Autodesk Fusion 360 part; units mm, degrees
(part 3 of 4)
  line L1272 (186.7093, 343.9871) -> (186.7093, 321.9621)
  line L1273 (186.7093, 321.9621) -> (208.7343, 321.9621)
  line L1274 (210.2343, 323.4621) -> (210.2343, 332.1121)
  line L1275 (210.2343, 332.1121) -> (213.3343, 332.1121)
  line L1276 (213.3343, 332.1121) -> (213.3343, 323.4621)
  line L1277 (214.8343, 321.9621) -> (236.8593, 321.9621)
  line L1278 (236.8593, 321.9621) -> (236.8593, 343.9871)
  line L1279 (235.3593, 345.4871) -> (226.7093, 345.4871)
  line L1280 (226.7093, 345.4871) -> (226.7093, 348.5871)
  line L1281 (226.7093, 348.5871) -> (235.3593, 348.5871)
  line L1282 (236.8593, 350.0871) -> (236.8593, 372.1121)
  line L1283 (236.8593, 372.1121) -> (214.8343, 372.1121)
  line L1284 (213.3343, 370.6121) -> (213.3343, 361.9621)
  line L1285 (213.3343, 361.9621) -> (210.2343, 361.9621)
  line L1286 (210.2343, 361.9621) -> (210.2343, 370.6121)
  line L1287 (208.7343, 372.1121) -> (186.7093, 372.1121)
  line L1288 (92.7953, 75.9662) -> (92.7953, 53.9412)
  line L1289 (94.2953, 52.4412) -> (102.9453, 52.4412)
  line L1290 (102.9453, 52.4412) -> (102.9453, 49.3412)
  line L1291 (102.9453, 49.3412) -> (94.2953, 49.3412)
  line L1292 (92.7953, 47.8412) -> (92.7953, 25.8162)
  line L1293 (92.7953, 25.8162) -> (114.8203, 25.8162)
  line L1294 (116.3203, 27.3162) -> (116.3203, 35.9662)
  line L1295 (116.3203, 35.9662) -> (119.4203, 35.9662)
  line L1296 (119.4203, 35.9662) -> (119.4203, 27.3162)
  line L1297 (120.9203, 25.8162) -> (142.9453, 25.8162)
  line L1298 (142.9453, 25.8162) -> (142.9453, 47.8412)
  line L1299 (141.4453, 49.3412) -> (132.7953, 49.3412)
  line L1300 (132.7953, 49.3412) -> (132.7953, 52.4412)
  line L1301 (132.7953, 52.4412) -> (141.4453, 52.4412)
  line L1302 (142.9453, 53.9412) -> (142.9453, 75.9662)
  line L1303 (142.9453, 75.9662) -> (120.9203, 75.9662)
  line L1304 (119.4203, 74.4662) -> (119.4203, 65.8162)
  line L1305 (119.4203, 65.8162) -> (116.3203, 65.8162)
  line L1306 (116.3203, 65.8162) -> (116.3203, 74.4662)
  line L1307 (114.8203, 75.9662) -> (92.7953, 75.9662)
  line L1308 (90.7952, 128.1162) -> (68.7702, 128.1162)
  line L1309 (67.2702, 126.6162) -> (67.2702, 117.9662)
  line L1310 (67.2702, 117.9662) -> (64.1702, 117.9662)
  line L1311 (64.1702, 117.9662) -> (64.1702, 126.6162)
  line L1312 (62.6702, 128.1162) -> (40.6452, 128.1162)
  line L1313 (40.6452, 128.1162) -> (40.6452, 106.0912)
  line L1314 (42.1452, 104.5912) -> (50.7952, 104.5912)
  line L1315 (50.7952, 104.5912) -> (50.7952, 101.4912)
  line L1316 (50.7952, 101.4912) -> (42.1452, 101.4912)
  line L1317 (40.6452, 99.9912) -> (40.6452, 77.9662)
  line L1318 (40.6452, 77.9662) -> (62.6702, 77.9662)
  line L1319 (64.1702, 79.4662) -> (64.1702, 88.1162)
  line L1320 (64.1702, 88.1162) -> (67.2702, 88.1162)
  line L1321 (67.2702, 88.1162) -> (67.2702, 79.4662)
  line L1322 (68.7702, 77.9662) -> (90.7952, 77.9662)
  line L1323 (90.7952, 77.9662) -> (90.7952, 99.9912)
  line L1324 (89.2952, 101.4912) -> (80.6452, 101.4912)
  line L1325 (80.6452, 101.4912) -> (80.6452, 104.5912)
  line L1326 (80.6452, 104.5912) -> (89.2952, 104.5912)
  line L1327 (90.7952, 106.0912) -> (90.7952, 128.1162)
  line L1328 (144.9453, 75.9662) -> (144.9453, 53.9412)
  line L1329 (146.4453, 52.4412) -> (155.0953, 52.4412)
  line L1330 (155.0953, 52.4412) -> (155.0953, 49.3412)
  line L1331 (155.0953, 49.3412) -> (146.4453, 49.3412)
  line L1332 (144.9453, 47.8412) -> (144.9453, 25.8162)
  line L1333 (144.9453, 25.8162) -> (166.9703, 25.8162)
  line L1334 (168.4703, 27.3162) -> (168.4703, 35.9662)
  line L1335 (168.4703, 35.9662) -> (171.5703, 35.9662)
  line L1336 (171.5703, 35.9662) -> (171.5703, 27.3162)
  line L1337 (173.0703, 25.8162) -> (195.0953, 25.8162)
  line L1338 (195.0953, 25.8162) -> (195.0953, 47.8412)
  line L1339 (193.5953, 49.3412) -> (184.9453, 49.3412)
  line L1340 (184.9453, 49.3412) -> (184.9453, 52.4412)
  line L1341 (184.9453, 52.4412) -> (193.5953, 52.4412)
  line L1342 (195.0953, 53.9412) -> (195.0953, 75.9662)
  line L1343 (195.0953, 75.9662) -> (173.0703, 75.9662)
  line L1344 (171.5703, 74.4662) -> (171.5703, 65.8162)
  line L1345 (171.5703, 65.8162) -> (168.4703, 65.8162)
  line L1346 (168.4703, 65.8162) -> (168.4703, 74.4662)
  line L1347 (166.9703, 75.9662) -> (144.9453, 75.9662)
  line L1348 (92.7953, 128.1162) -> (92.7953, 106.0912)
  line L1349 (94.2953, 104.5912) -> (102.9453, 104.5912)
  line L1350 (102.9453, 104.5912) -> (102.9453, 101.4912)
  line L1351 (102.9453, 101.4912) -> (94.2953, 101.4912)
  line L1352 (92.7953, 99.9912) -> (92.7953, 77.9662)
  line L1353 (92.7953, 77.9662) -> (114.8203, 77.9662)
  line L1354 (116.3203, 79.4662) -> (116.3203, 88.1162)
  line L1355 (116.3203, 88.1162) -> (119.4203, 88.1162)
  line L1356 (119.4203, 88.1162) -> (119.4203, 79.4662)
  line L1357 (120.9203, 77.9662) -> (142.9453, 77.9662)
  line L1358 (142.9453, 77.9662) -> (142.9453, 99.9912)
  line L1359 (141.4453, 101.4912) -> (132.7953, 101.4912)
  line L1360 (132.7953, 101.4912) -> (132.7953, 104.5912)
  line L1361 (132.7953, 104.5912) -> (141.4453, 104.5912)
  line L1362 (142.9453, 106.0912) -> (142.9453, 128.1162)
  line L1363 (142.9453, 128.1162) -> (120.9203, 128.1162)
  line L1364 (119.4203, 126.6162) -> (119.4203, 117.9662)
  line L1365 (119.4203, 117.9662) -> (116.3203, 117.9662)
  line L1366 (116.3203, 117.9662) -> (116.3203, 126.6162)
  line L1367 (114.8203, 128.1162) -> (92.7953, 128.1162)
  line L1368 (134.5593, 372.1123) -> (134.5593, 350.0873)
  line L1369 (136.0593, 348.5873) -> (144.7093, 348.5873)
  line L1370 (144.7093, 348.5873) -> (144.7093, 345.4873)
  line L1371 (144.7093, 345.4873) -> (136.0593, 345.4873)
  line L1372 (134.5593, 343.9873) -> (134.5593, 321.9623)
  line L1373 (134.5593, 321.9623) -> (156.5843, 321.9623)
  line L1374 (158.0843, 323.4623) -> (158.0843, 332.1123)
  line L1375 (158.0843, 332.1123) -> (161.1843, 332.1123)
  line L1376 (161.1843, 332.1123) -> (161.1843, 323.4623)
  line L1377 (162.6843, 321.9623) -> (184.7093, 321.9623)
  line L1378 (184.7093, 321.9623) -> (184.7093, 343.9873)
  line L1379 (183.2093, 345.4873) -> (174.5593, 345.4873)
  line L1380 (174.5593, 345.4873) -> (174.5593, 348.5873)
  line L1381 (174.5593, 348.5873) -> (183.2093, 348.5873)
  line L1382 (184.7093, 350.0873) -> (184.7093, 372.1123)
  line L1383 (184.7093, 372.1123) -> (162.6843, 372.1123)
  line L1384 (161.1843, 370.6123) -> (161.1843, 361.9623)
  line L1385 (161.1843, 361.9623) -> (158.0843, 361.9623)
  line L1386 (158.0843, 361.9623) -> (158.0843, 370.6123)
  line L1387 (156.5843, 372.1123) -> (134.5593, 372.1123)
  line L1388 (70.2592, 363.2374) -> (78.9092, 363.2374)
  line L1389 (80.4092, 364.7374) -> (80.4092, 374.2624)
  line L1390 (80.4092, 374.2624) -> (30.2592, 374.2624)
  line L1391 (30.2592, 374.2624) -> (30.2592, 364.7374)
  line L1392 (31.7592, 363.2374) -> (40.4092, 363.2374)
  line L1393 (40.4092, 363.2374) -> (40.4092, 360.1374)
  line L1394 (40.4092, 360.1374) -> (31.7592, 360.1374)
  line L1395 (30.2592, 358.6374) -> (30.2592, 349.1124)
  line L1396 (30.2592, 349.1124) -> (80.4092, 349.1124)
  line L1397 (80.4092, 349.1124) -> (80.4092, 358.6374)
  line L1398 (78.9092, 360.1374) -> (70.2592, 360.1374)
  line L1399 (70.2592, 360.1374) -> (70.2592, 363.2374)
  line L1400 (31.7593, 387.2874) -> (30.2593, 385.7874)
  line L1401 (80.4093, 385.7874) -> (78.9093, 387.2874)
  line L1402 (78.9093, 390.3874) -> (80.4093, 391.8874)
  line L1403 (30.2593, 391.8874) -> (31.7593, 390.3874)
  line L1404 (141.3991, 149.3871) -> (139.8991, 147.8871)
  line L1405 (190.0491, 147.8871) -> (188.5491, 149.3871)
  line L1406 (188.5491, 152.4871) -> (190.0491, 153.9871)
  line L1407 (139.8991, 153.9871) -> (141.3991, 152.4871)
  line L1408 (-15.1922, 249.7413) -> (-16.6922, 248.2413)
  line L1409 (33.4578, 248.2413) -> (31.9578, 249.7413)
  line L1410 (31.9578, 252.8413) -> (33.4578, 254.3413)
  line L1411 (-16.6922, 254.3413) -> (-15.1922, 252.8413)
  line L1412 (-15.0862, 168.2912) -> (-16.5862, 166.7912)
  line L1413 (33.5638, 166.7912) -> (32.0638, 168.2912)
  line L1414 (32.0638, 171.3912) -> (33.5638, 172.8912)
  line L1415 (-16.5862, 172.8912) -> (-15.0862, 171.3912)
  line L1416 (240.3594, 385.137) -> (238.8594, 383.637)
  line L1417 (289.0094, 383.637) -> (287.5094, 385.137)
  line L1418 (287.5094, 388.237) -> (289.0094, 389.737)
  line L1419 (238.8594, 389.737) -> (240.3594, 388.237)
  line L1420 (188.2094, 385.1371) -> (186.7094, 383.6371)
  line L1421 (236.8594, 383.6371) -> (235.3594, 385.1371)
  line L1422 (235.3594, 388.2371) -> (236.8594, 389.7371)
  line L1423 (186.7094, 389.7371) -> (188.2094, 388.2371)
  line L1424 (-29.576, 79.4662) -> (-28.076, 77.9662)
  line L1425 (-28.076, 128.1162) -> (-29.576, 126.6162)
  line L1426 (-32.676, 126.6162) -> (-34.176, 128.1162)
  line L1427 (-34.176, 77.9662) -> (-32.676, 79.4662)
  line L1428 (-32.7151, 178.7662) -> (-34.2151, 180.2662)
  line L1429 (-34.2151, 130.1162) -> (-32.7151, 131.6162)
  line L1430 (-29.6151, 131.6162) -> (-28.1151, 130.1162)
  line L1431 (-28.1151, 180.2662) -> (-29.6151, 178.7662)
  line L1432 (-24.5298, 27.3162) -> (-23.0298, 25.8162)
  line L1433 (-23.0298, 75.9662) -> (-24.5298, 74.4662)
  line L1434 (-27.6298, 74.4662) -> (-29.1298, 75.9662)
  line L1435 (-29.1298, 25.8162) -> (-27.6298, 27.3162)
  line L1436 (37.0991, 149.3873) -> (35.5991, 147.8873)
  line L1437 (85.7491, 147.8873) -> (84.2491, 149.3873)
  line L1438 (84.2491, 152.4873) -> (85.7491, 153.9873)
  line L1439 (35.5991, 153.9873) -> (37.0991, 152.4873)
  line L1440 (-20.3908, 304.0412) -> (-21.8908, 302.5412)
  line L1441 (28.2592, 302.5412) -> (26.7592, 304.0412)
  line L1442 (26.7592, 307.1412) -> (28.2592, 308.6412)
  line L1443 (-21.8908, 308.6412) -> (-20.3908, 307.1412)
  line L1444 (317.1876, 137.8303) -> (318.6876, 136.3303)
  line L1445 (318.6876, 186.4803) -> (317.1876, 184.9803)
  line L1446 (314.0876, 184.9803) -> (312.5876, 186.4803)
  line L1447 (312.5876, 136.3303) -> (314.0876, 137.8303)
  line L1448 (31.7592, 332.9874) -> (30.2592, 331.4874)
  line L1449 (80.4092, 331.4874) -> (78.9092, 332.9874)
  line L1450 (78.9092, 336.0874) -> (80.4092, 337.5874)
  line L1451 (30.2592, 337.5874) -> (31.7592, 336.0874)
  line L1452 (-15.1215, 195.4412) -> (-16.6215, 193.9412)
  line L1453 (33.5285, 193.9412) -> (32.0285, 195.4412)
  line L1454 (32.0285, 198.5412) -> (33.5285, 200.0412)
  line L1455 (-16.6215, 200.0412) -> (-15.1215, 198.5412)
  line L1456 (-15.1568, 222.5912) -> (-16.6568, 221.0912)
  line L1457 (33.4932, 221.0912) -> (31.9932, 222.5912)
  line L1458 (31.9932, 225.6912) -> (33.4932, 227.1912)
  line L1459 (-16.6568, 227.1912) -> (-15.1568, 225.6912)
  line L1460 (-20.3908, 385.491) -> (-21.8908, 383.991)
  line L1461 (28.2592, 383.991) -> (26.7592, 385.491)
  line L1462 (26.7592, 388.591) -> (28.2592, 390.091)
  line L1463 (-21.8908, 390.091) -> (-20.3908, 388.591)
  line L1464 (89.2491, 149.3871) -> (87.7491, 147.8871)
  line L1465 (137.8991, 147.8871) -> (136.3991, 149.3871)
  line L1466 (136.3991, 152.4871) -> (137.8991, 153.9871)
  line L1467 (87.7491, 153.9871) -> (89.2491, 152.4871)
  line L1468 (193.5491, 149.387) -> (192.0491, 147.887)
  line L1469 (242.1991, 147.887) -> (240.6991, 149.387)
  line L1470 (240.6991, 152.487) -> (242.1991, 153.987)
  line L1471 (192.0491, 153.987) -> (193.5491, 152.487)
  line L1472 (-15.051, 141.1412) -> (-16.551, 139.6412)
  line L1473 (33.599, 139.6412) -> (32.099, 141.1412)
  line L1474 (32.099, 144.2412) -> (33.599, 145.7412)
  line L1475 (-16.551, 145.7412) -> (-15.051, 144.2412)
  line L1476 (-20.3908, 276.8913) -> (-21.8908, 275.3913)
  line L1477 (28.2592, 275.3913) -> (26.7592, 276.8913)
  line L1478 (26.7592, 279.9913) -> (28.2592, 281.4913)
  line L1479 (-21.8908, 281.4913) -> (-20.3908, 279.9913)
  line L1480 (26.7592, 334.2911) -> (28.2592, 335.7911)
  line L1481 (-21.8908, 335.7911) -> (-20.3908, 334.2911)
  line L1482 (-20.3908, 331.1911) -> (-21.8908, 329.6911)
  line L1483 (28.2592, 329.6911) -> (26.7592, 331.1911)
  line L1484 (83.9094, 385.1373) -> (82.4094, 383.6373)
  line L1485 (132.5594, 383.6373) -> (131.0594, 385.1373)
  line L1486 (131.0594, 388.2373) -> (132.5594, 389.7373)
  line L1487 (82.4094, 389.7373) -> (83.9094, 388.2373)
  line L1488 (430.1484, 400.5165) -> (428.6484, 400.5165)
  line L1489 (425.9637, 402.0665) -> (425.2137, 403.3655)
  line L1490 (401.6433, 403.3655) -> (400.8933, 402.0665)
  line L1491 (398.2086, 400.5165) -> (396.7086, 400.5165)
  line L1492 (384.9234, 380.1039) -> (385.6734, 378.8048)
  line L1493 (385.6734, 375.7048) -> (384.9234, 374.4058)
  line L1494 (396.7086, 353.9932) -> (398.2086, 353.9932)
  line L1495 (400.8933, 352.4432) -> (401.6433, 351.1442)
  line L1496 (425.2137, 351.1442) -> (425.9637, 352.4432)
  line L1497 (428.6484, 353.9932) -> (430.1484, 353.9932)
  line L1498 (441.9336, 374.4058) -> (441.1836, 375.7048)
  line L1499 (441.1836, 378.8048) -> (441.9336, 380.1039)
  line L1500 (336.2343, 237.8526) -> (334.7343, 237.8526)
  line L1501 (332.0497, 239.4026) -> (331.2997, 240.7016)
  line L1502 (307.7292, 240.7016) -> (306.9792, 239.4026)
  line L1503 (304.2946, 237.8526) -> (302.7946, 237.8526)
  line L1504 (291.0093, 217.44) -> (291.7593, 216.1409)
  line L1505 (291.7593, 213.0409) -> (291.0093, 211.7419)
  line L1506 (302.7946, 191.3293) -> (304.2946, 191.3293)
  line L1507 (306.9792, 189.7793) -> (307.7292, 188.4803)
  line L1508 (331.2997, 188.4803) -> (332.0497, 189.7793)
  line L1509 (334.7343, 191.3293) -> (336.2343, 191.3293)
  line L1510 (348.0196, 211.7419) -> (347.2696, 213.0409)
  line L1511 (347.2696, 216.1409) -> (348.0196, 217.44)
  line L1512 (208.8805, 28.6652) -> (210.3805, 28.6652)
  line L1513 (213.0652, 27.1152) -> (213.8152, 25.8162)
  line L1514 (237.3856, 25.8162) -> (238.1356, 27.1152)
  line L1515 (240.8203, 28.6652) -> (242.3203, 28.6652)
  line L1516 (254.1055, 49.0778) -> (253.3555, 50.3768)
  line L1517 (253.3555, 53.4768) -> (254.1055, 54.7759)
  line L1518 (242.3203, 75.1885) -> (240.8203, 75.1885)
  line L1519 (238.1356, 76.7385) -> (237.3856, 78.0375)
  line L1520 (213.8152, 78.0375) -> (213.0652, 76.7385)
  line L1521 (210.3805, 75.1885) -> (208.8805, 75.1885)
  line L1522 (197.0953, 54.7759) -> (197.8453, 53.4768)
  line L1523 (197.8453, 50.3768) -> (197.0953, 49.0778)
  line L1524 (383.1914, 373.4056) -> (381.6914, 373.4056)
  line L1525 (379.0067, 374.9556) -> (378.2567, 376.2547)
  line L1526 (354.6863, 376.2547) -> (353.9363, 374.9556)
  line L1527 (351.2516, 373.4056) -> (349.7516, 373.4056)
  line L1528 (337.9664, 352.993) -> (338.7164, 351.694)
  line L1529 (338.7164, 348.594) -> (337.9664, 347.295)
  line L1530 (349.7516, 326.8824) -> (351.2516, 326.8824)
  line L1531 (353.9363, 325.3324) -> (354.6863, 324.0333)
  line L1532 (378.2567, 324.0333) -> (379.0067, 325.3324)
  line L1533 (381.6914, 326.8824) -> (383.1914, 326.8824)
  line L1534 (394.9766, 347.295) -> (394.2266, 348.594)
  line L1535 (394.2266, 351.694) -> (394.9766, 352.993)
  line L1536 (383.1914, 319.1845) -> (381.6914, 319.1845)
  line L1537 (379.0067, 320.7345) -> (378.2567, 322.0335)
  line L1538 (354.6863, 322.0335) -> (353.9363, 320.7345)
  line L1539 (351.2516, 319.1845) -> (349.7516, 319.1845)
  line L1540 (337.9664, 298.7719) -> (338.7164, 297.4729)
  line L1541 (338.7164, 294.3729) -> (337.9664, 293.0738)
  line L1542 (349.7516, 272.6613) -> (351.2516, 272.6613)
  line L1543 (353.9363, 271.1113) -> (354.6863, 269.8122)
  line L1544 (378.2567, 269.8122) -> (379.0067, 271.1113)
  line L1545 (381.6914, 272.6613) -> (383.1914, 272.6613)
  line L1546 (394.9766, 293.0738) -> (394.2266, 294.3729)
  line L1547 (394.2266, 297.4729) -> (394.9766, 298.7719)
  line L1548 (383.1913, 156.5205) -> (381.6913, 156.5205)
  line L1549 (379.0066, 158.0705) -> (378.2566, 159.3696)
  line L1550 (354.6862, 159.3696) -> (353.9362, 158.0705)
  line L1551 (351.2515, 156.5205) -> (349.7515, 156.5205)
  line L1552 (337.9663, 136.1079) -> (338.7163, 134.8089)
  line L1553 (338.7163, 131.7089) -> (337.9663, 130.4099)
  line L1554 (349.7515, 109.9973) -> (351.2515, 109.9973)
  line L1555 (353.9362, 108.4473) -> (354.6862, 107.1482)
  line L1556 (378.2566, 107.1482) -> (379.0066, 108.4473)
  line L1557 (381.6913, 109.9973) -> (383.1913, 109.9973)
  line L1558 (394.9765, 130.4099) -> (394.2265, 131.7089)
  line L1559 (394.2265, 134.8089) -> (394.9765, 136.1079)
  line L1560 (208.8805, 82.8866) -> (210.3805, 82.8866)
  line L1561 (213.0652, 81.3366) -> (213.8152, 80.0376)
  line L1562 (237.3856, 80.0376) -> (238.1356, 81.3366)
  line L1563 (240.8203, 82.8866) -> (242.3203, 82.8866)
  line L1564 (254.1055, 103.2992) -> (253.3555, 104.5982)
  line L1565 (253.3555, 107.6982) -> (254.1055, 108.9973)
  line L1566 (242.3203, 129.4099) -> (240.8203, 129.4099)
  line L1567 (238.1356, 130.9599) -> (237.3856, 132.2589)
  line L1568 (213.8152, 132.2589) -> (213.0652, 130.9599)
  line L1569 (210.3805, 129.4099) -> (208.8805, 129.4099)
  line L1570 (197.0953, 108.9973) -> (197.8453, 107.6982)
  line L1571 (197.8453, 104.5982) -> (197.0953, 103.2992)
  line L1572 (383.1913, 210.7418) -> (381.6913, 210.7418)
  line L1573 (379.0066, 212.2918) -> (378.2566, 213.5909)
  line L1574 (354.6862, 213.5909) -> (353.9362, 212.2918)
  line L1575 (351.2515, 210.7418) -> (349.7515, 210.7418)
  line L1576 (337.9663, 190.3292) -> (338.7163, 189.0302)
  line L1577 (338.7163, 185.9302) -> (337.9663, 184.6312)
  line L1578 (349.7515, 164.2186) -> (351.2515, 164.2186)
  line L1579 (353.9362, 162.6686) -> (354.6862, 161.3695)
  line L1580 (378.2566, 161.3695) -> (379.0066, 162.6686)
  line L1581 (381.6913, 164.2186) -> (383.1913, 164.2186)
  line L1582 (394.9765, 184.6312) -> (394.2265, 185.9302)
  line L1583 (394.2265, 189.0302) -> (394.9765, 190.3292)
  line L1584 (289.2773, 264.9631) -> (287.7773, 264.9631)
  line L1585 (285.0926, 266.5131) -> (284.3426, 267.8122)
  line L1586 (260.7722, 267.8122) -> (260.0222, 266.5131)
  line L1587 (257.3375, 264.9631) -> (255.8375, 264.9631)
  line L1588 (244.0523, 244.5505) -> (244.8023, 243.2515)
  line L1589 (244.8023, 240.1515) -> (244.0523, 238.8525)
  line L1590 (255.8375, 218.4399) -> (257.3375, 218.4399)
  line L1591 (260.0222, 216.8899) -> (260.7722, 215.5908)
  line L1592 (284.3426, 215.5908) -> (285.0926, 216.8899)
  line L1593 (287.7773, 218.4399) -> (289.2773, 218.4399)
  line L1594 (301.0625, 238.8525) -> (300.3125, 240.1515)
  line L1595 (300.3125, 243.2515) -> (301.0625, 244.5505)
  line L1596 (336.2343, 75.1885) -> (334.7343, 75.1885)
  line L1597 (332.0497, 76.7385) -> (331.2997, 78.0375)
  line L1598 (307.7292, 78.0375) -> (306.9792, 76.7385)
  line L1599 (304.2946, 75.1885) -> (302.7946, 75.1885)
  line L1600 (291.0093, 54.7759) -> (291.7593, 53.4769)
  line L1601 (291.7593, 50.3769) -> (291.0093, 49.0778)
  line L1602 (302.7946, 28.6652) -> (304.2946, 28.6652)
  line L1603 (306.9792, 27.1152) -> (307.7292, 25.8162)
  line L1604 (331.2997, 25.8162) -> (332.0497, 27.1152)
  line L1605 (334.7343, 28.6652) -> (336.2343, 28.6652)
  line L1606 (348.0196, 49.0778) -> (347.2696, 50.3769)
  line L1607 (347.2696, 53.4769) -> (348.0196, 54.7759)
  line L1608 (336.2345, 400.5165) -> (334.7345, 400.5165)
  line L1609 (332.0498, 402.0665) -> (331.2998, 403.3656)
  line L1610 (307.7294, 403.3656) -> (306.9794, 402.0665)
  line L1611 (304.2947, 400.5165) -> (302.7947, 400.5165)
  line L1612 (291.0095, 380.1039) -> (291.7595, 378.8049)
  line L1613 (291.7595, 375.7049) -> (291.0095, 374.4058)
  line L1614 (302.7947, 353.9933) -> (304.2947, 353.9933)
  line L1615 (306.9794, 352.4433) -> (307.7294, 351.1442)
  line L1616 (331.2998, 351.1442) -> (332.0498, 352.4433)
  line L1617 (334.7345, 353.9933) -> (336.2345, 353.9933)
  line L1618 (348.0197, 374.4058) -> (347.2697, 375.7049)
  line L1619 (347.2697, 378.8049) -> (348.0197, 380.1039)
  line L1620 (255.8376, 109.9972) -> (257.3376, 109.9972)
  line L1621 (260.0222, 108.4472) -> (260.7722, 107.1482)
  line L1622 (284.3427, 107.1482) -> (285.0927, 108.4472)
  line L1623 (287.7774, 109.9972) -> (289.2774, 109.9972)
  line L1624 (301.0626, 130.4098) -> (300.3126, 131.7088)
  line L1625 (300.3126, 134.8088) -> (301.0626, 136.1079)
  line L1626 (289.2774, 156.5205) -> (287.7774, 156.5205)
  line L1627 (285.0927, 158.0705) -> (284.3427, 159.3695)
  line L1628 (260.7722, 159.3695) -> (260.0222, 158.0705)
  line L1629 (257.3376, 156.5205) -> (255.8376, 156.5205)
  line L1630 (244.0524, 136.1079) -> (244.8024, 134.8088)
  line L1631 (244.8024, 131.7088) -> (244.0524, 130.4098)
  line L1632 (336.2343, 346.2952) -> (334.7343, 346.2952)
  line L1633 (332.0496, 347.8452) -> (331.2996, 349.1442)
  line L1634 (307.7292, 349.1442) -> (306.9792, 347.8452)
  line L1635 (304.2945, 346.2952) -> (302.7945, 346.2952)
  line L1636 (291.0093, 325.8826) -> (291.7593, 324.5836)
  line L1637 (291.7593, 321.4836) -> (291.0093, 320.1845)
  line L1638 (302.7945, 299.7719) -> (304.2945, 299.7719)
  line L1639 (306.9792, 298.2219) -> (307.7292, 296.9229)
  line L1640 (331.2996, 296.9229) -> (332.0496, 298.2219)
  line L1641 (334.7343, 299.7719) -> (336.2343, 299.7719)
  line L1642 (348.0195, 320.1845) -> (347.2695, 321.4836)
  line L1643 (347.2695, 324.5836) -> (348.0195, 325.8826)
  line L1644 (430.1484, 346.2951) -> (428.6484, 346.2951)
  line L1645 (425.9637, 347.8451) -> (425.2137, 349.1441)
  line L1646 (401.6433, 349.1441) -> (400.8933, 347.8451)
  line L1647 (398.2086, 346.2951) -> (396.7086, 346.2951)
  line L1648 (384.9234, 325.8825) -> (385.6734, 324.5835)
  line L1649 (385.6734, 321.4835) -> (384.9234, 320.1844)
  line L1650 (396.7086, 299.7719) -> (398.2086, 299.7719)
  line L1651 (400.8933, 298.2219) -> (401.6433, 296.9228)
  line L1652 (425.2137, 296.9228) -> (425.9637, 298.2219)
  line L1653 (428.6484, 299.7719) -> (430.1484, 299.7719)
  line L1654 (441.9336, 320.1844) -> (441.1836, 321.4835)
  line L1655 (441.1836, 324.5835) -> (441.9336, 325.8825)
  line L1656 (336.2343, 129.4099) -> (334.7343, 129.4099)
  line L1657 (332.0497, 130.9599) -> (331.2997, 132.2589)
  line L1658 (307.7292, 132.2589) -> (306.9792, 130.9599)
  line L1659 (304.2946, 129.4099) -> (302.7946, 129.4099)
  line L1660 (291.0093, 108.9973) -> (291.7593, 107.6982)
  line L1661 (291.7593, 104.5982) -> (291.0093, 103.2992)
  line L1662 (302.7946, 82.8866) -> (304.2946, 82.8866)
  line L1663 (306.9792, 81.3366) -> (307.7292, 80.0376)
  line L1664 (331.2997, 80.0376) -> (332.0497, 81.3366)
  line L1665 (334.7343, 82.8866) -> (336.2343, 82.8866)
  line L1666 (348.0196, 103.2992) -> (347.2696, 104.5982)
  line L1667 (347.2696, 107.6982) -> (348.0196, 108.9973)
  line L1668 (336.2343, 292.0738) -> (334.7343, 292.0738)
  line L1669 (332.0496, 293.6238) -> (331.2996, 294.9229)
  line L1670 (307.7292, 294.9229) -> (306.9792, 293.6238)
  line L1671 (304.2945, 292.0738) -> (302.7945, 292.0738)
  line L1672 (291.0093, 271.6612) -> (291.7593, 270.3622)
  line L1673 (291.7593, 267.2622) -> (291.0093, 265.9632)
  line L1674 (302.7945, 245.5506) -> (304.2945, 245.5506)
  line L1675 (306.9792, 244.0006) -> (307.7292, 242.7015)
  line L1676 (331.2996, 242.7015) -> (332.0496, 244.0006)
  line L1677 (334.7343, 245.5506) -> (336.2343, 245.5506)
  line L1678 (348.0195, 265.9632) -> (347.2695, 267.2622)
  line L1679 (347.2695, 270.3622) -> (348.0195, 271.6612)
  line L1680 (383.1914, 264.9632) -> (381.6914, 264.9632)
  line L1681 (379.0067, 266.5132) -> (378.2567, 267.8122)
  line L1682 (354.6863, 267.8122) -> (353.9363, 266.5132)
  line L1683 (351.2516, 264.9632) -> (349.7516, 264.9632)
  line L1684 (337.9664, 244.5506) -> (338.7164, 243.2515)
  line L1685 (338.7164, 240.1515) -> (337.9664, 238.8525)
  line L1686 (349.7516, 218.4399) -> (351.2516, 218.4399)
  line L1687 (353.9363, 216.8899) -> (354.6863, 215.5909)
  line L1688 (378.2567, 215.5909) -> (379.0067, 216.8899)
  line L1689 (381.6914, 218.4399) -> (383.1914, 218.4399)
  line L1690 (394.9766, 238.8525) -> (394.2266, 240.1515)
  line L1691 (394.2266, 243.2515) -> (394.9766, 244.5506)
  line L1692 (430.1484, 129.4099) -> (428.6484, 129.4099)
  line L1693 (425.9637, 130.9599) -> (425.2137, 132.2589)
  line L1694 (401.6433, 132.2589) -> (400.8933, 130.9599)
  line L1695 (398.2086, 129.4099) -> (396.7086, 129.4099)
  line L1696 (384.9234, 108.9973) -> (385.6734, 107.6982)
  line L1697 (385.6734, 104.5982) -> (384.9234, 103.2992)
  line L1698 (396.7086, 82.8866) -> (398.2086, 82.8866)
  line L1699 (400.8933, 81.3366) -> (401.6433, 80.0376)
  line L1700 (425.2137, 80.0376) -> (425.9637, 81.3366)
  line L1701 (428.6484, 82.8866) -> (430.1484, 82.8866)
  line L1702 (441.9336, 103.2992) -> (441.1836, 104.5982)
  line L1703 (441.1836, 107.6982) -> (441.9336, 108.9973)
  line L1704 (430.1484, 237.8525) -> (428.6484, 237.8525)
  line L1705 (425.9637, 239.4025) -> (425.2137, 240.7016)
  line L1706 (401.6433, 240.7016) -> (400.8933, 239.4025)
  line L1707 (398.2086, 237.8525) -> (396.7086, 237.8525)
  line L1708 (384.9234, 217.44) -> (385.6734, 216.1409)
  line L1709 (385.6734, 213.0409) -> (384.9234, 211.7419)
  line L1710 (396.7086, 191.3293) -> (398.2086, 191.3293)
  line L1711 (400.8933, 189.7793) -> (401.6433, 188.4802)
  line L1712 (425.2137, 188.4802) -> (425.9637, 189.7793)
  line L1713 (428.6484, 191.3293) -> (430.1484, 191.3293)
  line L1714 (441.9336, 211.7419) -> (441.1836, 213.0409)
  line L1715 (441.1836, 216.1409) -> (441.9336, 217.44)
  line L1716 (430.1484, 75.1885) -> (428.6484, 75.1885)
  line L1717 (425.9637, 76.7385) -> (425.2137, 78.0375)
  line L1718 (401.6433, 78.0375) -> (400.8933, 76.7385)
  line L1719 (398.2086, 75.1885) -> (396.7086, 75.1885)
  line L1720 (384.9234, 54.7759) -> (385.6734, 53.4769)
  line L1721 (385.6734, 50.3769) -> (384.9234, 49.0778)
  line L1722 (396.7086, 28.6652) -> (398.2086, 28.6652)
  line L1723 (400.8933, 27.1152) -> (401.6433, 25.8162)
  line L1724 (425.2137, 25.8162) -> (425.9637, 27.1152)
  line L1725 (428.6484, 28.6652) -> (430.1484, 28.6652)
  line L1726 (441.9336, 49.0778) -> (441.1836, 50.3769)
  line L1727 (441.1836, 53.4769) -> (441.9336, 54.7759)
  line L1728 (255.8378, 164.2185) -> (257.3378, 164.2185)
  line L1729 (260.0225, 162.6685) -> (260.7725, 161.3695)
  line L1730 (284.3429, 161.3695) -> (285.0929, 162.6685)
  line L1731 (287.7776, 164.2185) -> (289.2776, 164.2185)
  line L1732 (301.0628, 184.6311) -> (300.3128, 185.9302)
  line L1733 (300.3128, 189.0302) -> (301.0628, 190.3292)
  line L1734 (289.2776, 210.7418) -> (287.7776, 210.7418)
  line L1735 (285.0929, 212.2918) -> (284.3429, 213.5908)
  line L1736 (260.7725, 213.5908) -> (260.0225, 212.2918)
  line L1737 (257.3378, 210.7418) -> (255.8378, 210.7418)
  line L1738 (244.0526, 190.3292) -> (244.8026, 189.0302)
  line L1739 (244.8026, 185.9302) -> (244.0526, 184.6311)
  line L1740 (383.1913, 102.2992) -> (381.6913, 102.2992)
  line L1741 (379.0066, 103.8492) -> (378.2566, 105.1482)
  line L1742 (354.6862, 105.1482) -> (353.9362, 103.8492)
  line L1743 (351.2515, 102.2992) -> (349.7515, 102.2992)
  line L1744 (337.9663, 81.8866) -> (338.7163, 80.5875)
  line L1745 (338.7163, 77.4875) -> (337.9663, 76.1885)
  line L1746 (349.7515, 55.7759) -> (351.2515, 55.7759)
  line L1747 (353.9362, 54.2259) -> (354.6862, 52.9269)
  line L1748 (378.2566, 52.9269) -> (379.0066, 54.2259)
  line L1749 (381.6913, 55.7759) -> (383.1913, 55.7759)
  line L1750 (394.9765, 76.1885) -> (394.2265, 77.4875)
  line L1751 (394.2265, 80.5875) -> (394.9765, 81.8866)
  line L1752 (255.8376, 55.7759) -> (257.3376, 55.7759)
  line L1753 (260.0222, 54.2259) -> (260.7722, 52.9269)
  line L1754 (284.3427, 52.9269) -> (285.0927, 54.2259)
  line L1755 (287.7774, 55.7759) -> (289.2774, 55.7759)
  line L1756 (301.0626, 76.1885) -> (300.3126, 77.4876)
  line L1757 (300.3126, 80.5876) -> (301.0626, 81.8866)
  line L1758 (289.2774, 102.2992) -> (287.7774, 102.2992)
  line L1759 (285.0927, 103.8492) -> (284.3427, 105.1482)
  line L1760 (260.7722, 105.1482) -> (260.0222, 103.8492)
  line L1761 (257.3376, 102.2992) -> (255.8376, 102.2992)
  line L1762 (244.0524, 81.8866) -> (244.8024, 80.5876)
  line L1763 (244.8024, 77.4876) -> (244.0524, 76.1885)
  line L1764 (430.1484, 183.6312) -> (428.6484, 183.6312)
  line L1765 (425.9637, 185.1812) -> (425.2137, 186.4802)
  line L1766 (401.6433, 186.4802) -> (400.8933, 185.1812)
  line L1767 (398.2086, 183.6312) -> (396.7086, 183.6312)
  line L1768 (384.9234, 163.2186) -> (385.6734, 161.9196)
  line L1769 (385.6734, 158.8196) -> (384.9234, 157.5205)
  line L1770 (396.7086, 137.1079) -> (398.2086, 137.1079)
  line L1771 (400.8933, 135.5579) -> (401.6433, 134.2589)
  line L1772 (425.2137, 134.2589) -> (425.9637, 135.5579)
  line L1773 (428.6484, 137.1079) -> (430.1484, 137.1079)
  line L1774 (441.9336, 157.5205) -> (441.1836, 158.8196)
  line L1775 (441.1836, 161.9196) -> (441.9336, 163.2186)
  line L1776 (430.1484, 292.0739) -> (428.6484, 292.0739)
  line L1777 (425.9637, 293.6239) -> (425.2137, 294.9229)
  line L1778 (401.6433, 294.9229) -> (400.8933, 293.6239)
  line L1779 (398.2086, 292.0739) -> (396.7086, 292.0739)
  line L1780 (384.9234, 271.6613) -> (385.6734, 270.3622)
  line L1781 (385.6734, 267.2622) -> (384.9234, 265.9632)
  line L1782 (396.7086, 245.5506) -> (398.2086, 245.5506)
  line L1783 (400.8933, 244.0006) -> (401.6433, 242.7016)
  line L1784 (425.2137, 242.7016) -> (425.9637, 244.0006)
  line L1785 (428.6484, 245.5506) -> (430.1484, 245.5506)
  line L1786 (441.9336, 265.9632) -> (441.1836, 267.2622)
  line L1787 (441.1836, 270.3622) -> (441.9336, 271.6613)
  line L1788 (35.4525, 193.6374) -> (36.9525, 192.1374)
  line L1789 (36.9525, 189.0374) -> (35.4525, 187.5374)
  line L1790 (57.4775, 165.5124) -> (58.9775, 167.0124)
  line L1791 (62.0775, 167.0124) -> (63.5775, 165.5124)
  line L1792 (85.6025, 187.5374) -> (84.1025, 189.0374)
  line L1793 (84.1025, 192.1374) -> (85.6025, 193.6374)
  line L1794 (63.5775, 215.6624) -> (62.0775, 214.1624)
  line L1795 (58.9775, 214.1624) -> (57.4775, 215.6624)
  line L1796 (82.4091, 350.0873) -> (83.9091, 348.5873)
  line L1797 (83.9091, 345.4873) -> (82.4091, 343.9873)
  line L1798 (104.4341, 321.9623) -> (105.9341, 323.4623)
  line L1799 (109.0341, 323.4623) -> (110.5341, 321.9623)
  line L1800 (132.5591, 343.9873) -> (131.0591, 345.4873)
  line L1801 (131.0591, 348.5873) -> (132.5591, 350.0873)
  line L1802 (110.5341, 372.1123) -> (109.0341, 370.6123)
  line L1803 (105.9341, 370.6123) -> (104.4341, 372.1123)
  line L1804 (144.9454, 106.0912) -> (146.4454, 104.5912)
  line L1805 (146.4454, 101.4912) -> (144.9454, 99.9912)
  line L1806 (166.9704, 77.9662) -> (168.4704, 79.4662)
  line L1807 (171.5704, 79.4662) -> (173.0704, 77.9662)
  line L1808 (195.0954, 99.9912) -> (193.5954, 101.4912)
  line L1809 (193.5954, 104.5912) -> (195.0954, 106.0912)
  line L1810 (173.0704, 128.1162) -> (171.5704, 126.6162)
  line L1811 (168.4704, 126.6162) -> (166.9704, 128.1162)
  line L1812 (139.7525, 193.6371) -> (141.2525, 192.1371)
  line L1813 (141.2525, 189.0371) -> (139.7525, 187.5371)
  line L1814 (161.7775, 165.5121) -> (163.2775, 167.0121)
  line L1815 (166.3775, 167.0121) -> (167.8775, 165.5121)
  line L1816 (189.9025, 187.5371) -> (188.4025, 189.0371)
  line L1817 (188.4025, 192.1371) -> (189.9025, 193.6371)
  line L1818 (167.8775, 215.6621) -> (166.3775, 214.1621)
  line L1819 (163.2775, 214.1621) -> (161.7775, 215.6621)
  line L1820 (238.8593, 297.9372) -> (240.3593, 296.4372)
  line L1821 (240.3593, 293.3372) -> (238.8593, 291.8372)
  line L1822 (260.8843, 269.8122) -> (262.3843, 271.3122)
  line L1823 (265.4843, 271.3122) -> (266.9843, 269.8122)
  line L1824 (289.0093, 291.8372) -> (287.5093, 293.3372)
  line L1825 (287.5093, 296.4372) -> (289.0093, 297.9372)
  line L1826 (266.9843, 319.9622) -> (265.4843, 318.4622)
  line L1827 (262.3843, 318.4622) -> (260.8843, 319.9622)
  line L1828 (238.8594, 350.0872) -> (240.3594, 348.5872)
  line L1829 (240.3594, 345.4872) -> (238.8594, 343.9872)
  line L1830 (260.8844, 321.9622) -> (262.3844, 323.4622)
  line L1831 (265.4844, 323.4622) -> (266.9844, 321.9622)
  line L1832 (289.0094, 343.9872) -> (287.5094, 345.4872)
  line L1833 (287.5094, 348.5872) -> (289.0094, 350.0872)
  line L1834 (266.9844, 372.1122) -> (265.4844, 370.6122)
  line L1835 (262.3844, 370.6122) -> (260.8844, 372.1122)
  line L1836 (189.9026, 239.6871) -> (188.4026, 241.1871)
  line L1837 (188.4026, 244.2871) -> (189.9026, 245.7871)
  line L1838 (167.8776, 267.8121) -> (166.3776, 266.3121)
  line L1839 (163.2776, 266.3121) -> (161.7776, 267.8121)
  line L1840 (139.7526, 245.7871) -> (141.2526, 244.2871)
  line L1841 (141.2526, 241.1871) -> (139.7526, 239.6871)
  line L1842 (161.7776, 217.6621) -> (163.2776, 219.1621)
  line L1843 (166.3776, 219.1621) -> (167.8776, 217.6621)
  line L1844 (68.7702, 75.9662) -> (67.2702, 74.4662)
  line L1845 (64.1702, 74.4662) -> (62.6702, 75.9662)
  line L1846 (40.6452, 53.9412) -> (42.1452, 52.4412)
  line L1847 (42.1452, 49.3412) -> (40.6452, 47.8412)
  line L1848 (62.6702, 25.8162) -> (64.1702, 27.3162)
  line L1849 (67.2702, 27.3162) -> (68.7702, 25.8162)
  line L1850 (90.7952, 47.8412) -> (89.2952, 49.3412)
  line L1851 (89.2952, 52.4412) -> (90.7952, 53.9412)
  line L1852 (16.6202, 128.1161) -> (15.1202, 126.6161)
  line L1853 (12.0202, 126.6161) -> (10.5202, 128.1161)
  line L1854 (-11.5048, 106.0911) -> (-10.0048, 104.5911)
  line L1855 (-10.0048, 101.4911) -> (-11.5048, 99.9911)
  line L1856 (10.5202, 77.9661) -> (12.0202, 79.4661)
  line L1857 (15.1202, 79.4661) -> (16.6202, 77.9661)
  line L1858 (38.6452, 99.9911) -> (37.1452, 101.4911)
  line L1859 (37.1452, 104.5911) -> (38.6452, 106.0911)
  line L1860 (136.0594, 385.1371) -> (134.5594, 383.6371)
  line L1861 (184.7094, 383.6371) -> (183.2094, 385.1371)
  line L1862 (183.2094, 388.2371) -> (184.7094, 389.7371)
  line L1863 (134.5594, 389.7371) -> (136.0594, 388.2371)
  line L1864 (186.7093, 297.9371) -> (188.2093, 296.4371)
  line L1865 (188.2093, 293.3371) -> (186.7093, 291.8371)
  line L1866 (208.7343, 269.8121) -> (210.2343, 271.3121)
  line L1867 (213.3343, 271.3121) -> (214.8343, 269.8121)
  line L1868 (236.8593, 291.8371) -> (235.3593, 293.3371)
  line L1869 (235.3593, 296.4371) -> (236.8593, 297.9371)
  line L1870 (214.8343, 319.9621) -> (213.3343, 318.4621)
  line L1871 (210.2343, 318.4621) -> (208.7343, 319.9621)
  line L1872 (115.7275, 215.6625) -> (114.2275, 214.1625)
  line L1873 (111.1275, 214.1625) -> (109.6275, 215.6625)
  line L1874 (87.6025, 193.6375) -> (89.1025, 192.1375)
  line L1875 (89.1025, 189.0375) -> (87.6025, 187.5375)
  line L1876 (109.6275, 165.5125) -> (111.1275, 167.0125)
  line L1877 (114.2275, 167.0125) -> (115.7275, 165.5125)
  line L1878 (137.7525, 187.5375) -> (136.2525, 189.0375)
  line L1879 (136.2525, 192.1375) -> (137.7525, 193.6375)
  line L1880 (30.2591, 297.9374) -> (31.7591, 296.4374)
  line L1881 (31.7591, 293.3374) -> (30.2591, 291.8374)
  line L1882 (52.2841, 269.8124) -> (53.7841, 271.3124)
  line L1883 (56.8841, 271.3124) -> (58.3841, 269.8124)
  line L1884 (80.4091, 291.8374) -> (78.9091, 293.3374)
  line L1885 (78.9091, 296.4374) -> (80.4091, 297.9374)
  line L1886 (58.3841, 319.9624) -> (56.8841, 318.4624)
  line L1887 (53.7841, 318.4624) -> (52.2841, 319.9624)
  line L1888 (82.4091, 297.9374) -> (83.9091, 296.4374)
  line L1889 (83.9091, 293.3374) -> (82.4091, 291.8374)
  line L1890 (104.4341, 269.8124) -> (105.9341, 271.3124)
  line L1891 (109.0341, 271.3124) -> (110.5341, 269.8124)
  line L1892 (132.5591, 291.8374) -> (131.0591, 293.3374)
  line L1893 (131.0591, 296.4374) -> (132.5591, 297.9374)
  line L1894 (110.5341, 319.9624) -> (109.0341, 318.4624)
  line L1895 (105.9341, 318.4624) -> (104.4341, 319.9624)
  line L1896 (63.5777, 267.8124) -> (62.0777, 266.3124)
  line L1897 (58.9777, 266.3124) -> (57.4777, 267.8124)
  line L1898 (35.4527, 245.7874) -> (36.9527, 244.2874)
  line L1899 (36.9527, 241.1874) -> (35.4527, 239.6874)
  line L1900 (57.4777, 217.6624) -> (58.9777, 219.1624)
  line L1901 (62.0777, 219.1624) -> (63.5777, 217.6624)
  line L1902 (85.6027, 239.6874) -> (84.1027, 241.1874)
  line L1903 (84.1027, 244.2874) -> (85.6027, 245.7874)
  line L1904 (-11.5048, 53.9412) -> (-10.0048, 52.4412)
  line L1905 (-10.0048, 49.3412) -> (-11.5048, 47.8412)
  line L1906 (10.5202, 25.8162) -> (12.0202, 27.3162)
  line L1907 (15.1202, 27.3162) -> (16.6202, 25.8162)
  line L1908 (38.6452, 47.8412) -> (37.1452, 49.3412)
  line L1909 (37.1452, 52.4412) -> (38.6452, 53.9412)
  line L1910 (16.6202, 75.9662) -> (15.1202, 74.4662)
  line L1911 (12.0202, 74.4662) -> (10.5202, 75.9662)
  line L1912 (191.9024, 245.7871) -> (193.4024, 244.2871)
  line L1913 (193.4024, 241.1871) -> (191.9024, 239.6871)
  line L1914 (213.9274, 217.6621) -> (215.4274, 219.1621)
  line L1915 (218.5274, 219.1621) -> (220.0274, 217.6621)
  line L1916 (242.0524, 239.6871) -> (240.5524, 241.1871)
  line L1917 (240.5524, 244.2871) -> (242.0524, 245.7871)
  line L1918 (220.0274, 267.8121) -> (218.5274, 266.3121)
  line L1919 (215.4274, 266.3121) -> (213.9274, 267.8121)
  line L1920 (-20.3908, 358.3411) -> (-21.8908, 356.8411)
  line L1921 (28.2592, 356.8411) -> (26.7592, 358.3411)
  line L1922 (26.7592, 361.4411) -> (28.2592, 362.9411)
  line L1923 (-21.8908, 362.9411) -> (-20.3908, 361.4411)
  line L1924 (137.7527, 239.6874) -> (136.2527, 241.1874)
  line L1925 (136.2527, 244.2874) -> (137.7527, 245.7874)
  line L1926 (115.7277, 267.8124) -> (114.2277, 266.3124)
  line L1927 (111.1277, 266.3124) -> (109.6277, 267.8124)
  line L1928 (87.6027, 245.7874) -> (89.1027, 244.2874)
  line L1929 (89.1027, 241.1874) -> (87.6027, 239.6874)
  line L1930 (109.6277, 217.6624) -> (111.1277, 219.1624)
  line L1931 (114.2277, 219.1624) -> (115.7277, 217.6624)
  line L1932 (191.9024, 193.6371) -> (193.4024, 192.1371)
  line L1933 (193.4024, 189.0371) -> (191.9024, 187.5371)
  line L1934 (213.9274, 165.5121) -> (215.4274, 167.0121)
  line L1935 (218.5274, 167.0121) -> (220.0274, 165.5121)
  line L1936 (242.0524, 187.5371) -> (240.5524, 189.0371)
  line L1937 (240.5524, 192.1371) -> (242.0524, 193.6371)
  line L1938 (220.0274, 215.6621) -> (218.5274, 214.1621)
  line L1939 (215.4274, 214.1621) -> (213.9274, 215.6621)
  line L1940 (134.5592, 297.9373) -> (136.0592, 296.4373)
  line L1941 (136.0592, 293.3373) -> (134.5592, 291.8373)
  line L1942 (156.5842, 269.8123) -> (158.0842, 271.3123)
  line L1943 (161.1842, 271.3123) -> (162.6842, 269.8123)
  line L1944 (184.7092, 291.8373) -> (183.2092, 293.3373)
  line L1945 (183.2092, 296.4373) -> (184.7092, 297.9373)
  line L1946 (162.6842, 319.9623) -> (161.1842, 318.4623)
  line L1947 (158.0842, 318.4623) -> (156.5842, 319.9623)
  line L1948 (186.7093, 350.0871) -> (188.2093, 348.5871)
  line L1949 (188.2093, 345.4871) -> (186.7093, 343.9871)
  line L1950 (208.7343, 321.9621) -> (210.2343, 323.4621)
  line L1951 (213.3343, 323.4621) -> (214.8343, 321.9621)
  line L1952 (236.8593, 343.9871) -> (235.3593, 345.4871)
  line L1953 (235.3593, 348.5871) -> (236.8593, 350.0871)
  line L1954 (214.8343, 372.1121) -> (213.3343, 370.6121)
  line L1955 (210.2343, 370.6121) -> (208.7343, 372.1121)
  line L1956 (92.7953, 53.9412) -> (94.2953, 52.4412)
  line L1957 (94.2953, 49.3412) -> (92.7953, 47.8412)
  line L1958 (114.8203, 25.8162) -> (116.3203, 27.3162)
  line L1959 (119.4203, 27.3162) -> (120.9203, 25.8162)
  line L1960 (142.9453, 47.8412) -> (141.4453, 49.3412)
  line L1961 (141.4453, 52.4412) -> (142.9453, 53.9412)
  line L1962 (120.9203, 75.9662) -> (119.4203, 74.4662)
  line L1963 (116.3203, 74.4662) -> (114.8203, 75.9662)
  line L1964 (68.7702, 128.1162) -> (67.2702, 126.6162)
  line L1965 (64.1702, 126.6162) -> (62.6702, 128.1162)
  line L1966 (40.6452, 106.0912) -> (42.1452, 104.5912)
  line L1967 (42.1452, 101.4912) -> (40.6452, 99.9912)
  line L1968 (62.6702, 77.9662) -> (64.1702, 79.4662)
  line L1969 (67.2702, 79.4662) -> (68.7702, 77.9662)
  line L1970 (90.7952, 99.9912) -> (89.2952, 101.4912)
  line L1971 (89.2952, 104.5912) -> (90.7952, 106.0912)
  line L1972 (144.9453, 53.9412) -> (146.4453, 52.4412)
  line L1973 (146.4453, 49.3412) -> (144.9453, 47.8412)
  line L1974 (166.9703, 25.8162) -> (168.4703, 27.3162)
  line L1975 (171.5703, 27.3162) -> (173.0703, 25.8162)
  line L1976 (195.0953, 47.8412) -> (193.5953, 49.3412)
  line L1977 (193.5953, 52.4412) -> (195.0953, 53.9412)
  line L1978 (173.0703, 75.9662) -> (171.5703, 74.4662)
  line L1979 (168.4703, 74.4662) -> (166.9703, 75.9662)
  line L1980 (92.7953, 106.0912) -> (94.2953, 104.5912)
  line L1981 (94.2953, 101.4912) -> (92.7953, 99.9912)
  line L1982 (114.8203, 77.9662) -> (116.3203, 79.4662)
  line L1983 (119.4203, 79.4662) -> (120.9203, 77.9662)
  line L1984 (142.9453, 99.9912) -> (141.4453, 101.4912)
  line L1985 (141.4453, 104.5912) -> (142.9453, 106.0912)
  line L1986 (120.9203, 128.1162) -> (119.4203, 126.6162)
  line L1987 (116.3203, 126.6162) -> (114.8203, 128.1162)
  line L1988 (134.5593, 350.0873) -> (136.0593, 348.5873)
  line L1989 (136.0593, 345.4873) -> (134.5593, 343.9873)
  line L1990 (156.5843, 321.9623) -> (158.0843, 323.4623)
  line L1991 (161.1843, 323.4623) -> (162.6843, 321.9623)
  line L1992 (184.7093, 343.9873) -> (183.2093, 345.4873)
  line L1993 (183.2093, 348.5873) -> (184.7093, 350.0873)
  line L1994 (162.6843, 372.1123) -> (161.1843, 370.6123)
  line L1995 (158.0843, 370.6123) -> (156.5843, 372.1123)
  line L1996 (31.7592, 360.1374) -> (30.2592, 358.6374)
  line L1997 (80.4092, 358.6374) -> (78.9092, 360.1374)
  line L1998 (78.9092, 363.2374) -> (80.4092, 364.7374)
  line L1999 (30.2592, 364.7374) -> (31.7592, 363.2374)
component "Arrange1" placed x (1, 0, 0) y (0, 1, 0) z (0, 0, 1) at (0, 0, 0)
component "Component" placed x (1, 0, 0) y (0, 0, -1) z (0, 1, 0) at (5, 0, 406.2885)
component "Component'" placed x (0, 0, 1) y (1, 0, 0) z (0, 1, 0) at (303.2172, 0, -34.7628)
component "Component''" placed x (1, 0, 0) y (0, 0, -1) z (0, 1, 0) at (120.8462, 0, 416.6744)
component "Component'''" placed x (1, 0, 0) y (0, 0, -1) z (0, 1, 0) at (144.6963, 0, 434.3312)
component "Component''''" placed x (0, 0, 1) y (1, 0, 0) z (0, 1, 0) at (-5.3038, 0, 361.3312)
component "Component'''''" placed x (0, 0, 1) y (1, 0, 0) z (0, 1, 0) at (76.1461, 0, 314.3745)
component "Component''''''" placed x (0, 0, 1) y (1, 0, 0) z (0, 1, 0) at (-51.0038, 0, 314.3745)
component "Component'''''''" placed x (1, 0, 0) y (0, 0, -1) z (0, 1, 0) at (-217.85, 0, 406.2885)
component "Component''''''''" placed x (1, 0, 0) y (0, 0, -1) z (0, 1, 0) at (-78.1538, 0, 486.481)
component "Component'''''''''" placed x (0, 0, 1) y (1, 0, 0) z (0, 1, 0) at (-145, 0, 133.2885)
component "Component''''''''''" placed x (0, 0, 1) y (1, 0, 0) z (0, 1, 0) at (23.9962, 0, 91.5245)
component "Component'''''''''''" placed x (1, 0, 0) y (0, 0, -1) z (0, 1, 0) at (-217.85, 0, 758.4385)
component "Component''''''''''''" placed x (0, 0, 1) y (1, 0, 0) z (0, 1, 0) at (301.1461, 0, -287.7756)
component "Component'''''''''''''" placed x (0, 0, 1) y (1, 0, 0) z (0, 1, 0) at (-17.85, 0, -246.0116)
component "Component''''''''''''''" placed x (0, 0, 1) y (1, 0, 0) z (0, 1, 0) at (46.846, 0, -345.1187)
component "Component'''''''''''''''" placed x (0, 0, -1) y (-1, 0, 0) z (0, 1, 0) at (471.9962, 0, 909.3309)
component "Component''''''''''''''''" placed x (0, 0, 1) y (1, 0, 0) z (0, 1, 0) at (-155.304, 0, -345.1188)
component "Component'''''''''''''''''" placed x (0, 0, 1) y (1, 0, 0) z (0, 1, 0) at (248.9961, 0, -562.7756)
component "Component''''''''''''''''''" placed x (0, 0, 1) y (1, 0, 0) z (0, 1, 0) at (226.1459, 0, -614.9257)
component "Component'''''''''''''''''''" placed x (0, 0, 1) y (1, 0, 0) z (0, 1, 0) at (-145, 0, -521.0116)
component "Component''''''''''''''''''''" placed x (0, 0, 1) y (1, 0, 0) z (0, 1, 0) at (-220, 0, -573.1616)
component "Component'''''''''''''''''''''" placed x (0, 0, 1) y (1, 0, 0) z (0, 1, 0) at (-51.004, 0, -614.9257)
component "Component''''''''''''''''''''''" placed x (0, 0, -1) y (-1, 0, 0) z (0, 1, 0) at (246.9959, 0, 1407.181)
component "Component'''''''''''''''''''''''" placed x (0, 0, 1) y (1, 0, 0) z (0, 1, 0) at (173.996, 0, -942.0757)
component "Component''''''''''''''''''''''''" placed x (0, 0, 1) y (1, 0, 0) z (0, 1, 0) at (-92.85, 0, -848.1617)
component "Component'''''''''''''''''''''''''" placed x (0, 0, 1) y (1, 0, 0) z (0, 1, 0) at (76.146, 0, -942.0757)
component "Component''''''''''''''''''''''''''" placed x (0, 0, 1) y (1, 0, 0) z (0, 1, 0) at (-155.3041, 0, -842.9689)
component "Component'''''''''''''''''''''''''''" placed x (0, 0, 1) y (1, 0, 0) z (0, 1, 0) at (-15.7786, 0, 12.1942)
component "Component''''''''''''''''''''''''''''" placed x (0, 0, 1) y (1, 0, 0) z (0, 1, 0) at (98.996, 0, -34.7628)
component "Component'''''''''''''''''''''''''''''" placed x (0, 0, 1) y (1, 0, 0) z (0, 1, 0) at (-220, 0, 12.1942)
component "Component''''''''''''''''''''''''''''''" placed x (0, 0, 1) y (1, 0, 0) z (0, 1, 0) at (-105.2253, 0, -34.7628)
component "Component'''''''''''''''''''''''''''''''" placed x (0, 0, 1) y (1, 0, 0) z (0, 1, 0) at (330.328, 0, -356.7198)
component "Component''''''''''''''''''''''''''''''''" placed x (0, 0, 1) y (1, 0, 0) z (0, 1, 0) at (11.3321, 0, -309.7628)
component "Component'''''''''''''''''''''''''''''''''" placed x (0, 0, 1) y (1, 0, 0) z (0, 1, 0) at (-117.8893, 0, -309.7628)
component "Component''''''''''''''''''''''''''''''''''" placed x (0, 0, 1) y (1, 0, 0) z (0, 1, 0) at (-84.4466, 0, -309.7628)
component "Component'''''''''''''''''''''''''''''''''''" placed x (0, 0, 1) y (1, 0, 0) z (0, 1, 0) at (-23.8934, 0, -356.7198)
component "Component''''''''''''''''''''''''''''''''''''" placed x (0, 0, -1) y (-1, 0, 0) z (0, 1, 0) at (111.4427, 0, 886.5582)
component "Component'''''''''''''''''''''''''''''''''''''" placed x (0, 0, 1) y (1, 0, 0) z (0, 1, 0) at (92.6641, 0, -537.8058)
component "Component''''''''''''''''''''''''''''''''''''''" placed x (0, 0, -1) y (-1, 0, 0) z (0, 1, 0) at (234.332, 0, 839.6012)
component "Component'''''''''''''''''''''''''''''''''''''''" placed x (0, 0, 1) y (1, 0, 0) z (0, 1, 0) at (-3.1146, 0, -537.8057)
component "Component''''''''''''''''''''''''''''''''''''''''" placed x (0, 0, 1) y (1, 0, 0) z (0, 1, 0) at (-23.8933, 0, -537.8057)
component "Component'''''''''''''''''''''''''''''''''''''''''" placed x (0, 0, 1) y (1, 0, 0) z (0, 1, 0) at (194.7747, 0, -765.8488)
component "Component''''''''''''''''''''''''''''''''''''''''''" placed x (0, 0, -1) y (-1, 0, 0) z (0, 1, 0) at (132.2213, 0, 1161.5582)
component "Component'''''''''''''''''''''''''''''''''''''''''''" placed x (0, 0, -1) y (-1, 0, 0) z (0, 1, 0) at (342.7747, 0, 1114.601)
component "Component''''''''''''''''''''''''''''''''''''''''''''" placed x (0, 0, 1) y (1, 0, 0) z (0, 1, 0) at (105.328, 0, -812.806)
component "Component'''''''''''''''''''''''''''''''''''''''''''''" placed x (0, 0, -1) y (-1, 0, 0) z (0, 1, 0) at (438.5533, 0, 1114.6012)
component "Component''''''''''''''''''''''''''''''''''''''''''''''" placed x (0, 0, 1) y (1, 0, 0) z (0, 1, 0) at (59.2214, 0, -1181.7198)
component "Component'''''''''''''''''''''''''''''''''''''''''''''''" placed x (0, 0, 1) y (1, 0, 0) z (0, 1, 0) at (92.6641, 0, -1181.7198)
component "Component''''''''''''''''''''''''''''''''''''''''''''''''" placed x (0, 0, 1) y (1, 0, 0) z (0, 1, 0) at (71.8854, 0, -1181.7198)
component "Component'''''''''''''''''''''''''''''''''''''''''''''''''" placed x (0, 0, 1) y (1, 0, 0) z (0, 1, 0) at (-220, 0, -1181.7198)
component "Component''''''''''''''''''''''''''''''''''''''''''''''''''" placed x (0, 0, 1) y (1, 0, 0) z (0, 1, 0) at (-186.5573, 0, -1181.7198)
component "Component'''''''''''''''''''''''''''''''''''''''''''''''''''" placed x (1, 0, 0) y (0, 0, -1) z (0, 1, 0) at (147.9962, 0, 491.6744)
component "Component''''''''''''''''''''''''''''''''''''''''''''''''''''" placed x (0, 0, 1) y (1, 0, 0) z (0, 1, 0) at (-92.85, 0, 285.1847)
component "Component'''''''''''''''''''''''''''''''''''''''''''''''''''''" placed x (0, 0, 1) y (1, 0, 0) z (0, 1, 0) at (-220, 0, 280.1384)
component "Component''''''''''''''''''''''''''''''''''''''''''''''''''''''" placed x (0, 0, 1) y (1, 0, 0) z (0, 1, 0) at (-184.4859, 0, -61.579)
component "Component'''''''''''''''''''''''''''''''''''''''''''''''''''''''" placed x (1, 0, 0) y (0, 0, -1) z (0, 1, 0) at (-102.0039, 0, 364.5243)
component "Component''''''''''''''''''''''''''''''''''''''''''''''''''''''''" placed x (1, 0, 0) y (0, 0, -1) z (0, 1, 0) at (-337.7542, 0, 329.8845)
component "Component'''''''''''''''''''''''''''''''''''''''''''''''''''''''''" placed x (1, 0, 0) y (0, 0, -1) z (0, 1, 0) at (-264.5499, 0, 613.5905)
component "Component''''''''''''''''''''''''''''''''''''''''''''''''''''''''''" placed x (1, 0, 0) y (0, 0, -1) z (0, 1, 0) at (-346, 0, 688.4846)
component "Component'''''''''''''''''''''''''''''''''''''''''''''''''''''''''''" placed x (1, 0, 0) y (0, 0, -1) z (0, 1, 0) at (-291.7, 0, 763.5552)
component "Component''''''''''''''''''''''''''''''''''''''''''''''''''''''''''''" placed x (1, 0, 0) y (0, 0, -1) z (0, 1, 0) at (-377.0042, 0, 208.0742)
component "Component'''''''''''''''''''''''''''''''''''''''''''''''''''''''''''''" placed x (1, 0, 0) y (0, 0, -1) z (0, 1, 0) at (-612.7541, 0, 382.0345)
component "Component''''''''''''''''''''''''''''''''''''''''''''''''''''''''''''''" placed x (1, 0, 0) y (0, 0, -1) z (0, 1, 0) at (-512.3999, 0, 613.6259)
component "Component'''''''''''''''''''''''''''''''''''''''''''''''''''''''''''''''" placed x (1, 0, 0) y (0, 0, -1) z (0, 1, 0) at (-593.85, 0, 688.5199)
component "Component''''''''''''''''''''''''''''''''''''''''''''''''''''''''''''''''" placed x (1, 0, 0) y (0, 0, -1) z (0, 1, 0) at (-374.8538, 0, 716.6743)